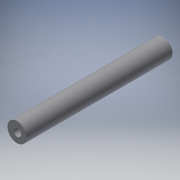
# Autodesk Inventor part: drive train standoff
Saved by Autodesk Inventor 2017 (Build 210142000, 142)
## iProperties
Created: 2017-07-19
Part Number: drive train standoff
Material: Generic
Document SubType Name: Modeling
Designer: User
Density: 1 g/cm^3
Appearance: Default
Mass: 5.46234 g
Surface Area: 28.2983 cm^2
Volume: 5.46234 cm^3
Author: User
Autodesk Inventor part; units mm, degrees
ref_plane "YZ Plane" through (0, 0, 0) normal (1, 0, 0) x (0, 1, 0)
ref_plane "XZ Plane" through (0, 0, 0) normal (0, 1, 0) x (-1, 0, 0)
ref_plane "XY Plane" through (0, 0, 0) normal (0, 0, 1) x (1, 0, 0)
sketch "Sketch1" plane through (0, 0, 0) normal (0, 0, 1) x (1, 0, 0)
  circle A0 centre (0, 0) radius 4.445
  dimension "d1" = 8.89
  constraints: 1 centre point, 1 coincident
  measures "d1" diameter of A0
extrude "Extrusion1" add sketch "Sketch1" along normal mid plane 90.6272
sketch "Sketch2" plane through (0, 0, 45.3136) normal (0, 0, 1) x (1, 0, 0)
  point P0 (0, 0)
hole "Hole1" at (0, 0, 45.3136) direction (0, 0, -1) diameter 3.683 depth 37.9984 tip angle 118 thread size "10-24 UNC" class "2B" standard "ANSI Unified Screw Threads"
thicken "Thicken1" operation add thickness 23.0632 both sides no extend neighbours yes toward (0, 0, -1) faces at (3.5296, -0.4286, 45.3136)
body "Solid1"
